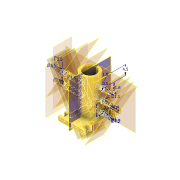
# Autodesk Inventor part: offset_cylinder
Saved by Autodesk Inventor 2021 (Build 250183000, 183)
## iProperties
Created: 2021-07-12
Part Number: offset_cylinder
Material: Generic
Document SubType Name: Modeling
Designer: Sihan
Density: 1 g/cm^3
Appearance: Default
Mass: 1.69832 g
Surface Area: 23.6767 cm^2
Volume: 1.69832 cm^3
Author: Sihan
Autodesk Inventor part; units mm, degrees
ref_plane "XZ Plane" through (0, 0, 0) normal (0, 1, 0) x (-1, 0, 0)
sketch "Sketch1" plane through (0, 0, 0) normal (0, 1, 0) x (-1, 0, 0)
  circle A0 centre (0, 0) radius 2.99
  circle A1 centre (0, 0) radius 4
  dimension "d0" = 5.98
  dimension "d1" = 8
  constraints: 2 centre point, 1 coincident
  measures "d0" diameter of A0
  measures "d1" diameter of A1
extrude "Extrusion1" add sketch "Sketch1" along normal blind 19
ref_plane "Work Plane1" through (6, 0, 0) normal (1, 0, 0) x (0, 1, 0)
sketch "Sketch2" plane through (6, 0, 0) normal (1, 0, 0) x (0, 1, 0)
  circle A0 centre (14.5, 0) radius 0.9
  circle A1 centre (9.5, 0) radius 0.9
  line L0 (19, -4) -> (19, 4) projected
  circle A2 centre (14.5, 0) radius 0.25
  circle A3 centre (9.5, 0) radius 0.25
  circle A4 centre (4.5, 0) radius 0.25
  circle A5 centre (4.5, 0) radius 0.9
  point P0 (0, 0)
  dimension "d5" = 1.8
  dimension "d7" = 1.8
  dimension "d9" = 4.5
  dimension "d16" = 0.5
  dimension "d18" = 0.5
  dimension "d82" = 5
  dimension "d144" = 0.5
  dimension "d145" = 1.8
  dimension "d152" = 5
  constraints: 6 centre point, 3 horizontal alignment, 1 coincident
  measures "d5" diameter of A0
  measures "d7" diameter of A1
  measures "d9" distance from line of L0 A0.centre
  measures "d16" diameter of A2
  measures "d18" diameter of A3
  measures "d82" distance of A1.centre A0.centre
  measures "d144" diameter of A4
  measures "d145" diameter of A5
  measures "d152" distance of A1.centre A5.centre
extrude "Extrusion2" add sketch "Sketch2" against normal up to next contours A0 | A1 | A2 | A3 | A4 | A5
extrude "Extrusion3" cut sketch "Sketch2" against normal up to next contours A2 | A3
sketch "Sketch3" plane through (0, 0, 0) normal (0, 0, 1) x (1, 0, 0)
  line L0 (6, 14.75) -> (6, 14.25) projected
  line L1 (6, 14.5) -> (10.9195, 14.5)
  line L2 (6, 14.5) -> (6, 15.6)
  line L3 (6, 15.6) -> (9.5, 15.2)
  line L4 (6, 9.75) -> (6, 9.25) projected
  line L5 (6, 9.5) -> (13.6368, 9.5)
  line L6 (6, 9.5) -> (6, 10.6)
  line L7 (6, 10.6) -> (9.5, 10.2)
  line L8 (9.5, 15.2) -> (9.5, 15.05)
  line L9 (9.5, 15.05) -> (6, 15.05)
  line L10 (9.5, 10.2) -> (9.5, 10)
  line L11 (9.5, 10) -> (6, 10)
  line L12 (6, 3.6) -> (6, 5.4) projected
  line L13 (6, 4.5) -> (13.6368, 4.5)
  line L14 (6, 4.5) -> (6, 5.6)
  line L15 (6, 5.6) -> (9.5, 5.2)
  line L16 (9.5, 5.2) -> (9.5, 5)
  line L17 (9.5, 5) -> (6, 5)
  point P0 (0, 0)
  point P1 (9.5, 7)
  dimension "d23" = 1.1
  dimension "d30" = 1.1
  dimension "d34" = 1.4
  dimension "d35" = 1.1
  dimension "d38" = 1.4
  dimension "d41" = 1
  dimension "d146" = 1
  dimension "d147" = 1.4
  dimension "d148" = 2.2
  dimension "d151" = 3.5
  constraints: 30 end point, 6 vertical, 4 midpoint, 3 horizontal, 3 perpendicular, 3 point on line
  measures "d23" distance of L1.start L2.end
  measures "d30" distance of L5.start L6.end
  measures "d34" diameter of L3.end L1
  measures "d35" diameter of L9 L1
  measures "d38" diameter of L7.end L5
  measures "d41" diameter of L11 L5
  measures "d146" diameter of L17 L13
  measures "d147" diameter of L15.end L13
  measures "d148" diameter of L14.end L13
  measures "d151" horizontal distance of L17.end L15.end
revolve "Revolution1" add sketch "Sketch3" angle 360 about axis through (6, 14.5, 0) along (1, 0, 0) separate body contours L2 L3 L8 L9
revolve "Revolution3" add sketch "Sketch3" angle 360 about axis through (6, 9.5, 0) along (1, 0, 0) separate body contours L6 L7 L10 L11
ref_plane "Work Plane2" through (0, 0, 0) normal (0.8660254, 0.5, 0) x (0, 0, 1)
ref_plane "Work Plane7" through (-13, 0, 0) normal (1, 0, 0) x (0, 1, 0)
sketch "Sketch4" plane through (-13, 0, 0) normal (1, 0, 0) x (0, 1, 0)
  circle A0 centre (12, 0) radius 0.9
  line L0 (19, -4) -> (19, 4) projected
  circle A1 centre (7, 0) radius 0.9
  line L1 (0, -4) -> (0, 4) projected
  point P0 (0, 0)
  dimension "d52" = 7
  dimension "d53" = 1.8
  dimension "d54" = 1.8
  dimension "d81" = 5
  constraints: 2 centre point
  measures "d52" distance from line of L0 A0.centre
  measures "d53" diameter of A0
  measures "d54" diameter of A1
  measures "d81" distance of A1.centre A0.centre
extrude "Extrusion4" add sketch "Sketch4" along normal up to next bodies 1
sketch "Sketch6" plane through (0, 0, 0) normal (0, 0, 1) x (1, 0, 0)
  line L0 (-13, 11.1) -> (-13, 12.9) projected
  line L1 (-13, 12) -> (-10.2091, 12)
  line L2 (-13, 12) -> (-13, 13.1)
  line L3 (-13, 13.1) -> (-16.5, 12.7)
  line L4 (-16.5, 12.7) -> (-16.5, 12.55)
  line L5 (-16.5, 12.55) -> (-13, 12.55)
  line L6 (-13, 6.1) -> (-13, 7.9) projected
  line L7 (-13, 7) -> (-10.2091, 7)
  line L8 (-13, 7) -> (-13, 8.1)
  line L9 (-13, 8.1) -> (-16.5, 7.7)
  line L10 (-16.5, 7.7) -> (-16.5, 7.55)
  line L11 (-16.5, 7.55) -> (-13, 7.55)
  point P0 (0, 0)
  point P1 (-13, 6.1)
  point P2 (-13, 7.9)
  dimension "d62" = 1.1
  dimension "d63" = 1.4
  dimension "d64" = 1.1
  dimension "d108" = 5
  dimension "d186" = 3.5
  constraints: 20 end point, 3 midpoint, 3 vertical, 1 horizontal, 1 perpendicular, 13 other
  measures "d62" diameter of L5 L1
  measures "d63" diameter of L3.end L1
  measures "d64" distance of L1.start L2.end
  measures "d108" distance of L1.start L7.start
  measures "d186" distance of L4.end L5.end
revolve "Revolution5" add sketch "Sketch6" angle 360 about axis through (-13, 12, 0) along (1, 0, 0) separate body contours L5 L4 L3 L2 L0
ref_plane "Work Plane8" through (0, 0, 0) normal (0.8660254, -0.5, 0) x (0, 0, 1)
ref_plane "Work Plane9" through (-9.1799, 5.3, 0) normal (0.8660254, -0.5, 0) x (0, 0, 1)
ref_plane "Work Plane10" through (-13.077, 7.55, 0) normal (0.8660254, -0.5, 0) x (0, 0, 1)
ref_plane "Work Plane14" through (-2.5981, -1.5, 0) normal (0.8660254, 0.5, 0) x (0, 0, 1)
ref_plane "Work Plane15" through (3.4641, -2, 0) normal (0.8660254, -0.5, 0) x (0, 0, 1)
ref_plane "Work Plane16" through (1.7321, -1, 0) normal (0.8660254, -0.5, 0) x (0, 0, 1)
pattern_of_nothing "Mirror1"
pattern_of_nothing "Mirror2"
revolve "Revolution9" add sketch "Sketch6" angle 360 about axis through (-13, 7, 0) along (1, 0, 0) separate body contours L11 L10 L9 L8 L6
ref_plane "Work Plane17" through (0, 0, -5) normal (0, 0, 1) x (1, 0, 0)
revolve "Revolution10" add sketch "Sketch3" angle 360 about axis through (6, 4.5, 0) along (1, 0, 0) separate body contours L12 L14 L15 L16 L17
ref_plane "Work Plane19" through (5.1962, -3, 0) normal (0.8660254, -0.5, 0) x (0, 0, 1)
ref_plane "Work Plane20" through (-4.3301, -2.5, 0) normal (0.8660254, 0.5, 0) x (0, 0, 1)
extrude "Extrusion13" cut sketch "Sketch2" against normal up to next contours A4 bodies 1
sketch "Sketch16" plane through (6, 14.5, 0) normal (1, 0, 0) x (0, 0, -1)
  circle A0 centre (0, 0) radius 0.5
  circle A1 centre (0, -10) radius 0.25 projected
  circle A2 centre (0, -5) radius 0.9 projected
  circle A3 centre (0, 0) radius 0.9 projected
  circle A4 centre (0, -5) radius 0.25 projected
  circle A5 centre (0, 0) radius 0.25 projected
  circle A6 centre (0, -10) radius 0.9 projected
  circle A7 centre (0, 0) radius 0.55 projected
  circle A8 centre (0, 0) radius 1.1 projected
  circle A9 centre (0, -5) radius 0.5 projected
  circle A10 centre (0, -5) radius 1.1 projected
  circle A11 centre (0, -10) radius 0.5 projected
  circle A12 centre (0, -10) radius 1.1 projected
  point P0 (0, -14.5)
  dimension "d156" = 1
  constraints: 1 centre point
  measures "d156" diameter of A0
extrude "Extrusion14" cut sketch "Sketch16" against normal up to surface contours A0 | A1 | A4 | A5 | A9 | A11 round surface about axis through (0, 0, 0) along (0, 1, 0) radius 2.99 far side no bodies 1
sketch "Sketch20" plane through (0, 0, 0) normal (0, -1, 0) x (1, 0, 0)
  line L0 (4, -9) -> (-4, -9)
  line L1 (-4, -9) -> (-4, 9)
  line L2 (-4, 9) -> (4, 9)
  line L3 (4, 9) -> (4, -9)
  line L4 (4, -9) -> (-4, 9) construction
  line L5 (-4, -9) -> (4, 9) construction
  circle A0 centre (0, 0) radius 4 projected
  point P0 (-4, 0)
  point P1 (4, 0)
  dimension "d174" = 8
  dimension "d175" = 18
  constraints: 12 end point, 2 midpoint, 2 parallel, 1 horizontal, 1 perpendicular
  measures "d174" distance of L1.end L2.end
  measures "d175" distance of L2.end L0.start
extrude "Extrusion18" add sketch "Sketch20" against normal blind 2 contours L0 L1 A0 L3 | A0 L1 L2 L3 bodies 1
sketch "Sketch21" plane through (4, 0, 9) normal (1, 0, 0) x (0, 0, -1)
  line L0 (0, 2) -> (18, 2) projected
  line L1 (18, 0) -> (0, 0) projected
  line L2 (0, 2) -> (1, 2)
  line L3 (1, 2) -> (1, 0)
  line L4 (1, 0) -> (0, 0)
  line L5 (0, 0) -> (0, 2)
  line L6 (3, 2) -> (4, 2)
  line L7 (4, 2) -> (4, 0)
  line L8 (4, 0) -> (3, 0)
  line L9 (3, 0) -> (3, 2)
  point P0 (9, 0)
  point P1 (8.7538, 2)
  point P2 (1, 2)
  dimension "d178" = 1
  dimension "d179" = 2
  dimension "d181" = 1
  constraints: 16 end point, 4 parallel, 3 point on line, 2 horizontal, 2 perpendicular
  measures "d178" distance between parallel lines of L3 L5
  measures "d179" distance between parallel lines of L9 L3
  measures "d181" distance between parallel lines of L9 L7
extrude "Extrusion19" add sketch "Sketch21" along normal blind 2 contours L0 L3 L1 L5 | L0 L7 L1 L9 bodies 1
mirror "Mirror4" about plane through (0, 0, 0) normal (0, 0, 1) of "Extrusion19" bodies 1
mirror "Mirror5" about plane through (0, 0, 0) normal (1, 0, 0) of "Extrusion19", "Mirror4" bodies 1
ref_plane "Work Plane21" through (-11, 0, 0) normal (1, 0, 0) x (0, 1, 0)
ref_plane "Work Plane11" through (0, 0, 0) normal (1, 0, 0) x (0, 1, 0)
fillet "Fillet5" radius 0.5 3 edges at (4, 13.6, -0.0018) (4, 8.6, -0.0018) (4, 3.6, -0.0018)
sketch "Sketch25" plane through (-11, 0, 0) normal (1, 0, 0) x (0, 1, 0)
  circle A0 centre (7, 0) radius 0.9 projected
  circle A1 centre (12, 0) radius 0.9 projected
  line L0 (12, 0) -> (7, 0) construction
  line L1 (12, 1.3) -> (7, 1.3)
  line L2 (7, -1.3) -> (12, -1.3)
  arc A2 (12, -1.3) -> (12, 1.3) centre (12, 0) ccw
  arc A3 (7, 1.3) -> (7, -1.3) centre (7, 0) ccw
  point P0 (0, 0)
  point P1 (9.5, 0)
  dimension "d194" = 1.3
  constraints: 8 end point, 4 point on circle, 4 tangent, 2 centre point, 1 horizontal, 1 midpoint, 1 parallel
  measures "d194" radius of A3
extrude "Extrusion23" add sketch "Sketch25" along normal up to surface contours A0 | A1 | A2 L2 A3 L1 round surface about axis through (0, 0, 0) along (0, 1, 0) radius 4 far side no bodies 1
sketch "Sketch24" plane through (-13, 12, 0) normal (-1, 0, 0) x (0, 0, 1)
  circle A0 centre (0, -5) radius 0.9 projected
  circle A1 centre (0, 0) radius 0.9 projected
  circle A2 centre (0, 0) radius 1.1 projected
  circle A3 centre (0, 0) radius 0.55 projected
  circle A4 centre (0, -5) radius 1.1 projected
  circle A5 centre (0, -5) radius 0.55 projected
  point P0 (0, -12)
extrude "Extrusion22" cut sketch "Sketch24" against normal up to surface contours A3 | A5 round surface about axis through (0, 0, 0) along (0, 1, 0) radius 2.99 far side no bodies 1
fillet "Fillet6" radius 0.5 2 edges at (-11, 11.1, 0) (-11, 6.1, 0)
ref_plane "Work Plane12" through (0, 0, 0) normal (-1, 0, 0) x (0, 1, 0)
ref_plane "Work Plane13" through (0, 0, 0) normal (-1, 0, 0) x (0, 1, 0)
body "Solid1"
body "Solid2"
body "Solid4"
body "Solid6"
body "Solid11"
body "Solid12"
